Autodesk Fusion 360 part; units mm, degrees
(part 5 of 7)
  spline S1395 degree 3 poles (51.3844, 45.9927) (51.2286, 46.0826) (51.0616, 46.1518) (50.8878, 46.1984) knots 0 0 0 0 1 1 1 1
  line L412 (26.6361, 48.608) -> (26.6361, 48.608)
  spline S1396 degree 3 poles (26.7927, 46.8149) (27.1126, 46.8435) (27.393, 47.0404) (27.5285, 47.3316) knots 0 0 0 0 1 1 1 1
  spline S1397 degree 3 poles (44.8618, 45.1809) (44.5277, 45.1809) (44.2072, 45.0481) (43.9709, 44.8119) knots 0 0 0 0 1 1 1 1
  spline S1398 degree 3 poles (52.4144, 44.2088) (52.4145, 44.3889) (52.3911, 44.5682) (52.3446, 44.7421) knots 0 0 0 0 1 1 1 1
  spline S1399 degree 3 poles (45.7533, 44.8119) (45.9895, 44.5756) (46.1222, 44.2551) (46.1222, 43.921) knots 0 0 0 0 1 1 1 1
  spline S1400 degree 3 poles (25.4878, 46.7012) (25.1676, 46.6732) (24.8568, 46.8182) (24.6724, 47.0815) knots 0 0 0 0 1 1 1 1
  line L413 (30.6519, 45.0444) -> (31.9567, 45.1586)
  spline S1401 degree 3 poles (24.6724, 47.0815) (24.8568, 46.8182) (25.1676, 46.6732) (25.4878, 46.7012) knots 0 0 0 0 1 1 1 1
  spline S1402 degree 3 poles (29.8359, 45.4253) (30.0203, 45.1616) (30.3314, 45.0164) (30.6519, 45.0444) knots 0 0 0 0 1 1 1 1
  spline S1403 degree 3 poles (50.8878, 46.1984) (50.7139, 46.245) (50.5346, 46.2686) (50.3545, 46.2686) knots 0 0 0 0 1 1 1 1
  spline S1404 degree 3 poles (26.6361, 48.608) (26.9561, 48.6355) (27.2664, 48.4904) (27.4505, 48.2272) knots 0 0 0 0 1 1 1 1
  spline S1405 degree 3 poles (52.3446, 44.7421) (52.2979, 44.916) (52.2285, 45.0829) (52.1384, 45.2387) knots 0 0 0 0 1 1 1 1
  spline S1406 degree 3 poles (43.9709, 44.8119) (43.7347, 44.5756) (43.602, 44.2551) (43.602, 43.921) knots 0 0 0 0 1 1 1 1
  spline S1407 degree 3 poles (43.9709, 43.0301) (43.7347, 43.2664) (43.602, 43.5868) (43.602, 43.921) knots 0 0 0 0 1 1 1 1
  spline S1408 degree 3 poles (43.602, 43.921) (43.602, 44.2551) (43.7347, 44.5756) (43.9709, 44.8119) knots 0 0 0 0 1 1 1 1
  spline S1409 degree 3 poles (108.6569, 74.2401) (108.9265, 73.999) (109.0957, 73.6656) (109.1313, 73.3057) knots 0 0 0 0 1 1 1 1
  line L414 (109.1313, 73.3057) -> (109.0982, 72.3565)
  line L415 (109.0982, 72.3565) -> (115.5945, 72.1296)
  line L416 (115.5945, 72.1296) -> (115.6275, 73.0789)
  line L417 (105.1589, 75.596) -> (106.0767, 74.6633)
  spline S1410 degree 3 poles (24.6724, 47.0815) (24.4883, 47.3449) (24.4585, 47.6864) (24.5944, 47.9776) knots 0 0 0 0 1 1 1 1
  line L418 (26.7927, 46.8149) -> (25.4878, 46.7012)
  spline S1411 degree 3 poles (32.6926, 45.6754) (32.8282, 45.9665) (32.7984, 46.3077) (32.6145, 46.571) knots 0 0 0 0 1 1 1 1
  line L419 (106.0767, 74.6633) -> (107.6761, 74.6075)
  line L420 (25.3307, 48.4938) -> (26.6361, 48.608)
  spline S1412 degree 3 poles (44.8618, 42.6611) (44.5277, 42.6611) (44.2072, 42.7938) (43.9709, 43.0301) knots 0 0 0 0 1 1 1 1
  spline S1413 degree 3 poles (27.4505, 48.2272) (27.2664, 48.4904) (26.9561, 48.6355) (26.6361, 48.608) knots 0 0 0 0 1 1 1 1
  spline S1414 degree 3 poles (29.7579, 46.3219) (29.6219, 46.0305) (29.6516, 45.6888) (29.8359, 45.4253) knots 0 0 0 0 1 1 1 1
  spline S1415 degree 3 poles (31.9567, 45.1586) (32.2766, 45.1872) (32.5571, 45.3842) (32.6926, 45.6754) knots 0 0 0 0 1 1 1 1
  spline S1416 degree 3 poles (63.315, 46.2438) (63.315, 46.578) (63.4477, 46.8984) (63.6839, 47.1347) knots 0 0 0 0 1 1 1 1
  spline S1417 degree 3 poles (32.6145, 46.571) (32.4305, 46.8341) (32.1201, 46.9793) (31.8001, 46.9518) knots 0 0 0 0 1 1 1 1
  spline S1418 degree 3 poles (51.8113, 45.6656) (51.6839, 45.7928) (51.5404, 45.9028) (51.3844, 45.9927) knots 0 0 0 0 1 1 1 1
  spline S1419 degree 3 poles (52.1384, 45.2387) (52.0485, 45.3947) (51.9385, 45.5382) (51.8113, 45.6656) knots 0 0 0 0 1 1 1 1
  line L421 (43.4733, 69.0828) -> (43.7141, 64.4892)
  line L422 (101.5374, 58.7118) -> (104.5657, 58.6064)
  line L423 (101.6982, 63.3095) -> (101.5374, 58.7118)
  line L424 (118.201, 72.989) -> (118.3612, 77.5866)
  spline S1420 degree 3 poles (107.0823, 57.6178) (107.4439, 57.6226) (107.7941, 57.4915) (108.0637, 57.2504) knots 0 0 0 0 1 1 1 1
  line L425 (110.2553, 62.51) -> (110.2904, 63.5094)
  line L426 (118.3612, 77.5866) -> (115.7877, 77.676)
  line L427 (110.8485, 79.4997) -> (110.8836, 80.4991)
  line L428 (115.2348, 61.8362) -> (110.7374, 61.9927)
  line L429 (46.0049, 69.6962) -> (46.0297, 69.2166)
  line L430 (115.828, 78.8258) -> (111.3306, 78.9824)
  line L431 (104.2561, 63.2201) -> (101.6982, 63.3095)
  spline S1421 degree 3 poles (107.6761, 74.6075) (108.0375, 74.6121) (108.3875, 74.481) (108.6569, 74.2401) knots 0 0 0 0 1 1 1 1
  line L432 (115.0343, 56.0892) -> (117.6078, 55.9998)
  line L433 (46.0297, 69.2166) -> (43.4733, 69.0828)
  line L434 (43.7141, 64.4892) -> (46.7398, 64.6474)
  line L435 (59.9596, 63.1875) -> (59.7188, 67.781)
  line L436 (46.7398, 64.6474) -> (47.7356, 63.7983)
  line L437 (110.2904, 63.5094) -> (109.8077, 64.0267)
  spline S1422 degree 3 poles (110.7374, 61.9927) (110.6043, 61.9961) (110.4782, 62.0529) (110.3875, 62.1504) knots 0 0 0 0 1 1 1 1
  line L438 (104.8111, 64.2014) -> (104.2732, 63.6996)
  line L439 (51.4899, 70.5044) -> (46.4969, 70.2424)
  line L440 (59.7188, 67.781) -> (57.1474, 67.6461)
  line L441 (50.8971, 62.7126) -> (50.9467, 61.7638)
  line L442 (102.1307, 75.7015) -> (105.1589, 75.596)
  spline S1423 degree 3 poles (49.3334, 63.882) (49.6932, 63.9184) (50.0535, 63.8185) (50.3432, 63.602) knots 0 0 0 0 1 1 1 1
  line L443 (52.0676, 69.0326) -> (52.0154, 70.031)
  line L444 (115.7877, 77.676) -> (115.828, 78.8258)
  spline S1424 degree 3 poles (50.3432, 63.602) (50.6327, 63.3853) (50.8304, 63.068) (50.8971, 62.7126) knots 0 0 0 0 1 1 1 1
  line L445 (105.4834, 57.6736) -> (107.0823, 57.6178)
  line L446 (115.0007, 55.1399) -> (115.0343, 56.0892)
  line L447 (47.7356, 63.7983) -> (49.3334, 63.882)
  line L448 (57.3882, 63.0526) -> (59.9596, 63.1875)
  line L449 (115.6275, 73.0789) -> (118.201, 72.989)
  spline S1425 degree 3 poles (52.5932, 68.5593) (52.4604, 68.5509) (52.3298, 68.5963) (52.2309, 68.6854) knots 0 0 0 0 1 1 1 1
  line L450 (57.1474, 67.6461) -> (57.0869, 68.7949)
  line L451 (52.3797, 53.5276) -> (47.3862, 53.2656)
  line L452 (52.0154, 70.031) -> (51.4899, 70.5044)
  spline S1426 degree 3 poles (52.2309, 68.6854) (52.132, 68.7744) (52.0731, 68.8996) (52.0676, 69.0326) knots 0 0 0 0 1 1 1 1
  line L453 (104.5657, 58.6064) -> (105.4834, 57.6736)
  line L454 (47.3862, 53.2656) -> (46.8943, 52.7194)
  line L455 (57.0869, 68.7949) -> (52.5932, 68.5593)
  line L456 (46.4969, 70.2424) -> (46.0049, 69.6962)
  line L457 (117.768, 60.597) -> (115.1945, 60.6869)
  line L458 (108.538, 56.3161) -> (108.505, 55.3668)
  spline S1427 degree 3 poles (111.3306, 78.9824) (111.1976, 78.9857) (111.0715, 79.0426) (110.9808, 79.14) knots 0 0 0 0 1 1 1 1
  line L459 (110.8836, 80.4991) -> (110.401, 81.0164)
  line L460 (115.1945, 60.6869) -> (115.2348, 61.8362)
  line L461 (108.505, 55.3668) -> (115.0007, 55.1399)
  spline S1428 degree 3 poles (110.3875, 62.1504) (110.2969, 62.2476) (110.2493, 62.3772) (110.2553, 62.51) knots 0 0 0 0 1 1 1 1
  line L462 (110.401, 81.0164) -> (105.4044, 81.1911)
  line L463 (104.2732, 63.6996) -> (104.2561, 63.2201)
  line L464 (109.8077, 64.0267) -> (104.8111, 64.2014)
  line L465 (57.4378, 62.1039) -> (57.3882, 63.0526)
  line L466 (50.9467, 61.7638) -> (57.4378, 62.1039)
  spline S1429 degree 3 poles (110.9808, 79.14) (110.8902, 79.2373) (110.8425, 79.3669) (110.8485, 79.4997) knots 0 0 0 0 1 1 1 1
  line L467 (117.6078, 55.9998) -> (117.768, 60.597)
  spline S1430 degree 3 poles (108.0637, 57.2504) (108.3332, 57.0094) (108.5025, 56.6759) (108.538, 56.3161) knots 0 0 0 0 1 1 1 1
  line L468 (60.849, 46.2108) -> (60.6082, 50.8043)
  line L469 (52.3797, 53.5276) -> (52.9053, 53.0543)
  line L470 (44.604, 47.5125) -> (47.6296, 47.6706)
  spline S1431 degree 3 poles (52.9575, 52.0559) (52.963, 51.9229) (53.0218, 51.7977) (53.1208, 51.7086) knots 0 0 0 0 1 1 1 1
  line L471 (52.9053, 53.0543) -> (52.9575, 52.0559)
  line L472 (50.2233, 46.9053) -> (48.6254, 46.8216)
  spline S1432 degree 3 poles (51.2325, 46.6252) (50.943, 46.8416) (50.5829, 46.9416) (50.2233, 46.9053) knots 0 0 0 0 1 1 1 1
  line L473 (25.9297, 42.6239) -> (26.3307, 38.0412)
  line L474 (30.3738, 37.4919) -> (31.9681, 37.6315)
  line L475 (29.3491, 38.3053) -> (30.3738, 37.4919)
  line L476 (60.6082, 50.8043) -> (60.849, 46.2108)
  line L477 (28.438, 43.3252) -> (28.4799, 42.8472)
  line L478 (33.892, 44.3246) -> (28.9109, 43.8884)
  line L479 (48.6254, 46.8216) -> (47.6296, 47.6706)
  line L480 (28.4799, 42.8472) -> (25.9297, 42.6239)
  line L481 (47.3862, 53.2656) -> (52.3797, 53.5276)
  line L482 (47.6296, 47.6706) -> (44.604, 47.5125)
  line L483 (46.8943, 52.7194) -> (47.3862, 53.2656)
  line L484 (51.8361, 44.7871) -> (51.7865, 45.7359)
  line L485 (40.0461, 37.0832) -> (42.6113, 37.3074)
  line L486 (44.3632, 52.106) -> (46.9196, 52.2399)
  line L487 (42.6113, 37.3074) -> (42.2108, 41.8901)
  line L488 (33.6537, 35.5701) -> (40.1293, 36.137)
  line L489 (26.3307, 38.0412) -> (29.3491, 38.3053)
  line L490 (39.6456, 41.6658) -> (39.5454, 42.8115)
  line L491 (39.5454, 42.8115) -> (35.0624, 42.4193)
  spline S1433 degree 3 poles (35.0624, 42.4193) (34.9301, 42.4062) (34.798, 42.447) (34.6961, 42.5324) knots 0 0 0 0 1 1 1 1
  spline S1434 degree 3 poles (34.6961, 42.5324) (34.5942, 42.618) (34.5311, 42.7409) (34.5209, 42.8735) knots 0 0 0 0 1 1 1 1
  line L492 (34.4335, 43.8698) -> (33.892, 44.3246)
  spline S1435 degree 3 poles (50.2233, 46.9053) (50.5829, 46.9416) (50.943, 46.8416) (51.2325, 46.6252) knots 0 0 0 0 1 1 1 1
  line L493 (58.2776, 46.0759) -> (60.849, 46.2108)
  line L494 (52.9053, 53.0543) -> (52.3797, 53.5276)
  line L495 (58.0367, 50.6694) -> (60.6082, 50.8043)
  line L496 (58.3272, 45.1271) -> (51.8361, 44.7871)
  line L497 (44.604, 47.5125) -> (44.3632, 52.106)
  line L498 (28.9109, 43.8884) -> (28.438, 43.3252)
  line L499 (46.9196, 52.2399) -> (46.8943, 52.7194)
  spline S1436 degree 3 poles (51.7865, 45.7359) (51.7197, 46.0912) (51.522, 46.4086) (51.2325, 46.6252) knots 0 0 0 0 1 1 1 1
  line L500 (57.9768, 51.8182) -> (53.483, 51.5825)
  spline S1437 degree 3 poles (31.9681, 37.6315) (32.3263, 37.6801) (32.6898, 37.5925) (32.9866, 37.386) knots 0 0 0 0 1 1 1 1
  line L501 (40.1293, 36.137) -> (40.0461, 37.0832)
  line L502 (44.3632, 52.106) -> (44.604, 47.5125)
  line L503 (33.5711, 36.5168) -> (33.6537, 35.5701)
  spline S1438 degree 3 poles (32.9866, 37.386) (33.2834, 37.1796) (33.4919, 36.8695) (33.5711, 36.5168) knots 0 0 0 0 1 1 1 1
  line L504 (34.5209, 42.8735) -> (34.4335, 43.8698)
  spline S1439 degree 3 poles (51.2325, 46.6252) (51.522, 46.4086) (51.7197, 46.0912) (51.7865, 45.7359) knots 0 0 0 0 1 1 1 1
  line L505 (58.2776, 46.0759) -> (58.3272, 45.1271)
  line L506 (51.7865, 45.7359) -> (51.8361, 44.7871)
  line L507 (52.9575, 52.0559) -> (52.9053, 53.0543)
  spline S1440 degree 3 poles (53.1208, 51.7086) (53.2197, 51.6196) (53.3502, 51.5742) (53.483, 51.5825) knots 0 0 0 0 1 1 1 1
  spline S1441 degree 3 poles (53.1208, 51.7086) (53.0218, 51.7977) (52.963, 51.9229) (52.9575, 52.0559) knots 0 0 0 0 1 1 1 1
  line L508 (53.483, 51.5825) -> (57.9768, 51.8182)
  line L509 (42.2108, 41.8901) -> (39.6456, 41.6658)
  line L510 (46.9196, 52.2399) -> (44.3632, 52.106)
  line L511 (51.8361, 44.7871) -> (58.3272, 45.1271)
  line L512 (58.0367, 50.6694) -> (57.9768, 51.8182)
  line L513 (60.849, 46.2108) -> (58.2776, 46.0759)
  line L514 (57.9768, 51.8182) -> (58.0367, 50.6694)
  spline S1442 degree 3 poles (53.483, 51.5825) (53.3502, 51.5742) (53.2197, 51.6196) (53.1208, 51.7086) knots 0 0 0 0 1 1 1 1
  line L515 (46.8943, 52.7194) -> (46.9196, 52.2399)
  line L516 (48.6254, 46.8216) -> (50.2233, 46.9053)
  line L517 (47.6296, 47.6706) -> (48.6254, 46.8216)
  line L518 (60.6082, 50.8043) -> (58.0367, 50.6694)
  line L519 (58.3272, 45.1271) -> (58.2776, 46.0759)
  line L520 (82.8492, 51.5396) -> (82.7686, 46.9404)
  spline S1443 degree 3 poles (73.2301, 53.5886) (73.136, 53.6826) (73.0836, 53.8106) (73.0849, 53.9436) knots 0 0 0 0 1 1 1 1
  line L521 (91.4192, 50.8901) -> (91.4363, 51.8895)
  line L522 (85.417, 51.9748) -> (85.4087, 51.4947)
  line L523 (80.6602, 52.2936) -> (78.0851, 52.2936)
  line L524 (101.1044, 46.3198) -> (100.9442, 41.7227)
  line L525 (78.0851, 46.7436) -> (78.0851, 47.6934)
  line L526 (72.5852, 55.4438) -> (67.585, 55.4438)
  line L527 (100.9442, 41.7227) -> (103.9724, 41.6167)
  line L528 (114.4075, 38.1503) -> (114.441, 39.0996)
  line L529 (117.1747, 43.6073) -> (114.6012, 43.6972)
  line L530 (114.6012, 43.6972) -> (114.6415, 44.8465)
  line L531 (85.7984, 46.8872) -> (86.7327, 45.971)
  line L532 (85.9461, 52.4858) -> (85.417, 51.9748)
  line L533 (104.8902, 40.684) -> (106.4891, 40.6282)
  line L534 (103.6799, 46.71) -> (103.6629, 46.2304)
  line L535 (67.0651, 54.4439) -> (64.5051, 54.4439)
  line L536 (73.0849, 54.9436) -> (72.5852, 55.4438)
  line L537 (64.5051, 49.8436) -> (67.5349, 49.8436)
  line L538 (64.5051, 54.4439) -> (64.5051, 49.8436)
  line L539 (71.5853, 46.7436) -> (78.0851, 46.7436)
  line L540 (78.0851, 53.4434) -> (73.5851, 53.4434)
  line L541 (78.0851, 52.2936) -> (78.0851, 53.4434)
  line L542 (86.7327, 45.971) -> (88.332, 45.9431)
  line L543 (89.81, 44.6672) -> (89.7935, 43.7174)
  spline S1444 degree 3 poles (91.5577, 50.5325) (91.4653, 50.6282) (91.4154, 50.7571) (91.4192, 50.8901) knots 0 0 0 0 1 1 1 1
  line L544 (103.6629, 46.2304) -> (101.1044, 46.3198)
  line L545 (104.2179, 47.2117) -> (103.6799, 46.71)
  line L546 (107.9117, 38.3771) -> (114.4075, 38.1503)
  spline S1445 degree 3 poles (106.4891, 40.6282) (106.8507, 40.6329) (107.2009, 40.5018) (107.4704, 40.2607) knots 0 0 0 0 1 1 1 1
  spline S1446 degree 3 poles (107.4704, 40.2607) (107.74, 40.0197) (107.9093, 39.6863) (107.9448, 39.3264) knots 0 0 0 0 1 1 1 1
  line L547 (98.964, 49.1077) -> (96.3894, 49.1527)
  line L548 (114.441, 39.0996) -> (117.014, 39.0102)
  spline S1447 degree 3 poles (110.1441, 45.0036) (110.0112, 45.0068) (109.8851, 45.0634) (109.7943, 45.1607) knots 0 0 0 0 1 1 1 1
  line L549 (85.4087, 51.4947) -> (82.8492, 51.5396)
  line L550 (68.4852, 48.9434) -> (70.0851, 48.9434)
  line L551 (82.7686, 46.9404) -> (85.7984, 46.8872)
  line L552 (71.5853, 47.6934) -> (71.5853, 46.7436)
  spline S1448 degree 3 poles (88.332, 45.9431) (88.6935, 45.9541) (89.0459, 45.8291) (89.3196, 45.5927) knots 0 0 0 0 1 1 1 1
  spline S1449 degree 3 poles (89.3196, 45.5927) (89.5931, 45.3565) (89.7681, 45.0262) (89.81, 44.6672) knots 0 0 0 0 1 1 1 1
  line L553 (103.9724, 41.6167) -> (104.8902, 40.684)
  line L554 (107.9448, 39.3264) -> (107.9117, 38.3771)
  line L555 (117.014, 39.0102) -> (117.1747, 43.6073)
  line L556 (109.6966, 46.5198) -> (109.2145, 47.0371)
  line L557 (67.0651, 54.9234) -> (67.0651, 54.4439)
  line L558 (96.2928, 43.6037) -> (96.3093, 44.5535)
  line L559 (96.4096, 50.3025) -> (91.9101, 50.3811)
  line L560 (90.9453, 52.3985) -> (85.9461, 52.4858)
  spline S1450 degree 3 poles (71.0783, 48.6106) (71.3562, 48.3792) (71.5371, 48.0518) (71.5853, 47.6934) knots 0 0 0 0 1 1 1 1
  spline S1451 degree 3 poles (91.9101, 50.3811) (91.7771, 50.3821) (91.65, 50.4367) (91.5577, 50.5325) knots 0 0 0 0 1 1 1 1
  line L561 (89.7935, 43.7174) -> (96.2928, 43.6037)
  line L562 (96.3093, 44.5535) -> (98.8839, 44.5085)
  spline S1452 degree 3 poles (109.7943, 45.1607) (109.7037, 45.258) (109.656, 45.3876) (109.662, 45.5204) knots 0 0 0 0 1 1 1 1
  line L563 (91.4363, 51.8895) -> (90.9453, 52.3985)
  line L564 (96.3894, 49.1527) -> (96.4096, 50.3025)
  line L565 (73.0849, 53.9436) -> (73.0849, 54.9436)
  line L566 (67.585, 55.4438) -> (67.0651, 54.9234)
  line L567 (98.8839, 44.5085) -> (98.964, 49.1077)
  line L568 (80.6602, 47.6934) -> (80.6602, 52.2936)
  line L569 (109.2145, 47.0371) -> (104.2179, 47.2117)
  spline S1453 degree 3 poles (70.0851, 48.9434) (70.4462, 48.9607) (70.8006, 48.842) (71.0783, 48.6106) knots 0 0 0 0 1 1 1 1
  line L570 (67.5349, 49.8436) -> (68.4852, 48.9434)
  line L571 (78.0851, 47.6934) -> (80.6602, 47.6934)
  spline S1454 degree 3 poles (73.5851, 53.4434) (73.4521, 53.4421) (73.3241, 53.4944) (73.2301, 53.5886) knots 0 0 0 0 1 1 1 1
  line L572 (96.3217, 22.9538) -> (97.0829, 21.8893)
  spline S1455 degree 3 poles (95.2588, 76.2513) (95.495, 76.4876) (95.6277, 76.8081) (95.6277, 77.1422) knots 0 0 0 0 1 1 1 1
  line L573 (95.5197, 77.6223) -> (93.3219, 77.661)
  line L574 (110.7958, 18.1474) -> (111.035, 17.4518)
  line L575 (109.662, 45.5204) -> (109.6966, 46.5198)
  line L576 (118.23, 26.2037) -> (117.1959, 26.7081)
  line L577 (111.035, 17.4518) -> (111.4665, 17.2415)
  line L578 (122.3641, 24.1873) -> (123.4932, 26.5019)
  line L579 (94.2252, 28.0475) -> (93.3478, 23.5321)
  spline S1456 degree 3 poles (100.2342, 85.5541) (99.906, 85.226) (99.7216, 84.781) (99.7215, 84.317) knots 0 0 0 0 1 1 1 1
  spline S1457 degree 3 poles (114.5547, 22.4329) (114.6738, 22.3733) (114.8118, 22.3642) (114.9377, 22.4076) knots 0 0 0 0 1 1 1 1
  line L580 (111.035, 17.4518) -> (110.7958, 18.1474)
  line L581 (120.3688, 17.9288) -> (123.2183, 23.7708)
  line L582 (93.3478, 23.5321) -> (96.3217, 22.9538)
  line L583 (96.7383, 27.5592) -> (94.2252, 28.0475)
  line L584 (114.5547, 22.4329) -> (113.6561, 22.8716)
  line L585 (112.9874, 22.6412) -> (113.6561, 22.8716)
  spline S1458 degree 3 poles (100.2342, 83.0793) (100.5624, 82.751) (101.0076, 82.5666) (101.4718, 82.5667) knots 0 0 0 0 1 1 1 1
  line L586 (110.7958, 18.1474) -> (112.9874, 22.6412)
  spline S1459 degree 3 poles (115.2234, 22.6634) (115.1664, 22.5432) (115.0634, 22.451) (114.9377, 22.4076) knots 0 0 0 0 1 1 1 1
  line L587 (111.4665, 17.2415) -> (110.3441, 14.9409)
  line L588 (117.1959, 26.7081) -> (115.2234, 22.6634)
  line L589 (110.3441, 14.9409) -> (111.4665, 17.2415)
  line L590 (110.3441, 14.9409) -> (114.4788, 12.9239)
  spline S1460 degree 3 poles (114.9377, 22.4076) (114.8118, 22.3642) (114.6738, 22.3733) (114.5547, 22.4329) knots 0 0 0 0 1 1 1 1
  line L591 (114.4788, 12.9239) -> (110.3441, 14.9409)
  line L592 (115.8068, 15.6473) -> (114.4788, 12.9239)
  line L593 (113.6561, 22.8716) -> (114.5547, 22.4329)
  spline S1461 degree 3 poles (101.9245, 86.0073) (101.7768, 86.0468) (101.6247, 86.0668) (101.4718, 86.0667) knots 0 0 0 0 1 1 1 1
  spline S1462 degree 3 poles (102.3467, 85.8321) (102.2142, 85.9087) (102.0723, 85.9676) (101.9245, 86.0073) knots 0 0 0 0 1 1 1 1
  line L594 (111.4665, 17.2415) -> (111.035, 17.4518)
  line L595 (123.2183, 23.7708) -> (122.3641, 24.1873)
  line L596 (97.4395, 28.4413) -> (96.8297, 28.03)
  spline S1463 degree 3 poles (95.6277, 77.1422) (95.6276, 77.2745) (95.6067, 77.406) (95.5657, 77.5318) knots 0 0 0 0 1 1 1 1
  line L597 (113.6561, 22.8716) -> (112.9874, 22.6412)
  line L598 (119.5146, 18.3453) -> (120.3688, 17.9288)
  line L599 (112.9874, 22.6412) -> (110.7958, 18.1474)
  spline S1464 degree 3 poles (118.4687, 18.2916) (118.7983, 18.4398) (119.1716, 18.4589) (119.5146, 18.3453) knots 0 0 0 0 1 1 1 1
  line L600 (97.0829, 21.8893) -> (98.6534, 21.5839)
  spline S1465 degree 3 poles (101.4718, 82.5667) (101.9358, 82.5668) (102.3808, 82.7512) (102.7089, 83.0793) knots 0 0 0 0 1 1 1 1
  spline S1466 degree 3 poles (99.7215, 84.317) (99.7215, 83.8527) (99.9059, 83.4075) (100.2342, 83.0793) knots 0 0 0 0 1 1 1 1
  line L601 (123.4932, 26.5019) -> (119.3586, 28.5183)
  spline S1467 degree 3 poles (102.7089, 83.0793) (103.0372, 83.4075) (103.2216, 83.8527) (103.2216, 84.317) knots 0 0 0 0 1 1 1 1
  spline S1468 degree 3 poles (117.7339, 17.5448) (117.8767, 17.877) (118.1389, 18.1434) (118.4687, 18.2916) knots 0 0 0 0 1 1 1 1
  spline S1469 degree 3 poles (101.4718, 86.0667) (101.0076, 86.0668) (100.5624, 85.8824) (100.2342, 85.5541) knots 0 0 0 0 1 1 1 1
  spline S1470 degree 3 poles (103.2216, 84.317) (103.2216, 84.4698) (103.2016, 84.622) (103.1621, 84.7696) knots 0 0 0 0 1 1 1 1
  spline S1471 degree 3 poles (98.6534, 21.5839) (98.7952, 21.5632) (98.9331, 21.5216) (99.0627, 21.4603) knots 0 0 0 0 1 1 1 1
  spline S1472 degree 3 poles (95.5657, 77.5318) (95.5516, 77.5626) (95.5363, 77.5928) (95.5197, 77.6223) knots 0 0 0 0 1 1 1 1
  spline S1473 degree 3 poles (99.0627, 21.4603) (99.1921, 21.3993) (99.3117, 21.3194) (99.4177, 21.2232) knots 0 0 0 0 1 1 1 1
  spline S1474 degree 3 poles (102.9875, 85.1918) (102.9109, 85.3242) (102.8172, 85.446) (102.7089, 85.5541) knots 0 0 0 0 1 1 1 1
  spline S1475 degree 3 poles (103.1621, 84.7696) (103.1226, 84.9174) (103.0639, 85.0593) (102.9875, 85.1918) knots 0 0 0 0 1 1 1 1
  line L602 (104.8499, 80.2097) -> (102.2914, 80.2991)
  line L603 (114.6415, 44.8465) -> (110.1441, 45.0036)
  spline S1476 degree 3 poles (102.7089, 85.5541) (102.6009, 85.6622) (102.4791, 85.7557) (102.3467, 85.8321) knots 0 0 0 0 1 1 1 1
  line L604 (105.4044, 81.1911) -> (104.8664, 80.6893)
  line L605 (114.4788, 12.9239) -> (115.8068, 15.6473)
  line L606 (115.8068, 15.6473) -> (117.0321, 16.1067)
  line L607 (104.8664, 80.6893) -> (104.8499, 80.2097)
  line L608 (102.2914, 80.2991) -> (102.1307, 75.7015)
  spline S1477 degree 3 poles (94.3679, 75.8823) (94.702, 75.8823) (95.0225, 76.015) (95.2588, 76.2513) knots 0 0 0 0 1 1 1 1
  line L609 (101.4718, 86.0667) -> (101.4718, 86.0667)
  line L610 (119.3586, 28.5183) -> (118.23, 26.2037)
  line L611 (117.0321, 16.1067) -> (117.7339, 17.5448)
  line L612 (96.8297, 28.03) -> (96.7383, 27.5592)
  spline S1478 degree 3 poles (121.6039, 11.6785) (121.2832, 11.6562) (120.9988, 11.4645) (120.8577, 11.1757) knots 0 0 0 0 1 1 1 1
  spline S1479 degree 3 poles (121.6039, 11.6785) (121.63, 11.6804) (121.6563, 11.681) (121.6825, 11.6806) knots 0 0 0 0 1 1 1 1
  line L613 (106.0865, 17.8978) -> (99.706, 19.138)
  line L614 (109.6734, 22.8546) -> (108.7954, 18.3391)
  line L615 (115.2234, 22.6634) -> (117.1959, 26.7081)
  line L616 (99.706, 19.138) -> (99.8874, 20.0708)
  spline S1480 degree 3 poles (132.2467, 31.0722) (132.379, 30.9957) (132.5008, 30.9022) (132.6089, 30.7941) knots 0 0 0 0 1 1 1 1
  line L617 (118.23, 26.2037) -> (119.3586, 28.5183)
  line L618 (108.7954, 18.3391) -> (106.2679, 18.8305)
  spline S1481 degree 3 poles (114.9377, 22.4076) (115.0634, 22.451) (115.1664, 22.5432) (115.2234, 22.6634) knots 0 0 0 0 1 1 1 1
  line L619 (102.9477, 25.3335) -> (107.365, 24.4746)
  line L620 (121.9016, 9.2094) -> (122.4757, 10.3866)
  spline S1482 degree 3 poles (121.1554, 8.7076) (121.4758, 8.7298) (121.7602, 8.921) (121.9016, 9.2094) knots 0 0 0 0 1 1 1 1
  spline S1483 degree 3 poles (131.8245, 31.2473) (131.9723, 31.2077) (132.1142, 31.1488) (132.2467, 31.0722) knots 0 0 0 0 1 1 1 1
  spline S1484 degree 3 poles (99.8487, 20.4961) (99.8148, 20.6353) (99.7605, 20.7687) (99.6874, 20.8919) knots 0 0 0 0 1 1 1 1
  spline S1485 degree 3 poles (99.8874, 20.0708) (99.8956, 20.2137) (99.8826, 20.357) (99.8487, 20.4961) knots 0 0 0 0 1 1 1 1
  line L621 (125.6832, 15.2519) -> (125.6832, 15.2519)
  line L622 (94.2252, 28.0475) -> (96.7383, 27.5592)
  line L623 (117.7339, 17.5448) -> (117.0321, 16.1067)
  line L624 (117.1959, 26.7081) -> (118.23, 26.2037)
  line L625 (121.6039, 11.6785) -> (121.6039, 11.6785)
  spline S1486 degree 3 poles (120.3477, 9.1014) (120.1677, 9.3676) (120.1433, 9.7095) (120.2836, 9.9985) knots 0 0 0 0 1 1 1 1
  spline S1487 degree 3 poles (132.6089, 30.7941) (132.7172, 30.6861) (132.8108, 30.5643) (132.8875, 30.4319) knots 0 0 0 0 1 1 1 1
  line L626 (124.3629, 13.5719) -> (124.937, 14.7491)
  line L627 (102.743, 26.9014) -> (102.5524, 25.9195)
  spline S1488 degree 3 poles (102.5524, 25.9195) (102.5256, 25.7892) (102.5524, 25.6536) (102.6268, 25.5433) knots 0 0 0 0 1 1 1 1
  spline S1489 degree 3 poles (102.6268, 25.5433) (102.7012, 25.4331) (102.8169, 25.3575) (102.9477, 25.3335) knots 0 0 0 0 1 1 1 1
  spline S1490 degree 3 poles (99.4177, 21.2232) (99.3117, 21.3194) (99.1921, 21.3993) (99.0627, 21.4603) knots 0 0 0 0 1 1 1 1
  line L628 (120.8577, 11.1757) -> (120.2836, 9.9985)
  spline S1491 degree 3 poles (120.2836, 9.9985) (120.1433, 9.7095) (120.1677, 9.3676) (120.3477, 9.1014) knots 0 0 0 0 1 1 1 1
  spline S1492 degree 3 poles (133.0621, 30.0097) (133.1016, 29.862) (133.1216, 29.7099) (133.1215, 29.557) knots 0 0 0 0 1 1 1 1
  spline S1493 degree 3 poles (99.6874, 20.8919) (99.6144, 21.0151) (99.5235, 21.1267) (99.4177, 21.2232) knots 0 0 0 0 1 1 1 1
  line L629 (122.4757, 10.3866) -> (121.9016, 9.2094)
  line L630 (97.0829, 21.8893) -> (96.3217, 22.9538)
  line L631 (120.2836, 9.9985) -> (120.8577, 11.1757)
  spline S1494 degree 3 poles (118.4687, 18.2916) (118.1389, 18.1434) (117.8767, 17.877) (117.7339, 17.5448) knots 0 0 0 0 1 1 1 1
  spline S1495 degree 3 poles (132.8875, 30.4319) (132.9639, 30.2994) (133.0226, 30.1575) (133.0621, 30.0097) knots 0 0 0 0 1 1 1 1
  spline S1496 degree 3 poles (120.3477, 9.1014) (120.5274, 8.8355) (120.8352, 8.6855) (121.1554, 8.7076) knots 0 0 0 0 1 1 1 1
  spline S1497 degree 3 poles (121.9016, 9.2094) (121.7602, 8.921) (121.4758, 8.7298) (121.1554, 8.7076) knots 0 0 0 0 1 1 1 1
  line L632 (102.3477, 27.4874) -> (102.743, 26.9014)
  line L633 (93.3478, 23.5321) -> (94.2252, 28.0475)
  line L634 (96.3217, 22.9538) -> (93.3478, 23.5321)
  line L635 (98.6534, 21.5839) -> (97.0829, 21.8893)
  spline S1498 degree 3 poles (99.0627, 21.4603) (98.9331, 21.5216) (98.7952, 21.5632) (98.6534, 21.5839) knots 0 0 0 0 1 1 1 1
  spline S1499 degree 3 poles (124.937, 14.7491) (125.0781, 15.038) (125.3626, 15.2296) (125.6832, 15.2519) knots 0 0 0 0 1 1 1 1
  line L636 (121.6825, 11.6806) -> (121.6825, 11.6806)
  line L637 (107.1454, 23.346) -> (109.6734, 22.8546)
  line L638 (119.3586, 28.5183) -> (123.4932, 26.5019)
  line L639 (96.8297, 28.03) -> (97.4395, 28.4413)
  line L640 (122.3641, 24.1873) -> (123.2183, 23.7708)
  line L641 (96.7383, 27.5592) -> (96.8297, 28.03)
  spline S1500 degree 3 poles (125.2347, 12.2816) (124.9147, 12.2596) (124.6072, 12.4096) (124.4275, 12.6754) knots 0 0 0 0 1 1 1 1
  spline S1501 degree 3 poles (122.4126, 11.2842) (122.5925, 11.0178) (122.6165, 10.6756) (122.4757, 10.3866) knots 0 0 0 0 1 1 1 1
  spline S1502 degree 3 poles (124.4275, 12.6754) (124.2476, 12.9413) (124.223, 13.283) (124.3629, 13.5719) knots 0 0 0 0 1 1 1 1
  line L642 (107.365, 24.4746) -> (107.1454, 23.346)
  spline S1503 degree 3 poles (122.4757, 10.3866) (122.6165, 10.6756) (122.5925, 11.0178) (122.4126, 11.2842) knots 0 0 0 0 1 1 1 1
  line L643 (117.0321, 16.1067) -> (115.8068, 15.6473)
  spline S1504 degree 3 poles (121.6825, 11.6806) (121.9759, 11.6754) (122.2484, 11.5275) (122.4126, 11.2842) knots 0 0 0 0 1 1 1 1
  spline S1505 degree 3 poles (121.1554, 8.7076) (120.8352, 8.6855) (120.5274, 8.8355) (120.3477, 9.1014) knots 0 0 0 0 1 1 1 1
  spline S1506 degree 3 poles (120.8577, 11.1757) (120.9988, 11.4645) (121.2832, 11.6562) (121.6039, 11.6785) knots 0 0 0 0 1 1 1 1
  spline S1507 degree 3 poles (131.3718, 31.3068) (131.5246, 31.3068) (131.6768, 31.2868) (131.8245, 31.2473) knots 0 0 0 0 1 1 1 1
  line L644 (106.2679, 18.8305) -> (106.0865, 17.8978)
  spline S1508 degree 3 poles (122.4126, 11.2842) (122.2328, 11.5506) (121.9246, 11.7009) (121.6039, 11.6785) knots 0 0 0 0 1 1 1 1
  line L645 (97.4395, 28.4413) -> (102.3477, 27.4874)
  line L646 (70.73, 75.2436) -> (69.42, 75.2436)
  line L647 (64.5051, 66.8436) -> (67.5349, 66.8436)
  spline S1509 degree 3 poles (122.9563, 22.4939) (123.0821, 22.4531) (123.2007, 22.3927) (123.3077, 22.3151) knots 0 0 0 0 1 1 1 1
  spline S1510 degree 3 poles (119.5146, 18.3453) (119.1716, 18.4589) (118.7983, 18.4398) (118.4687, 18.2916) knots 0 0 0 0 1 1 1 1
  spline S1511 degree 3 poles (121.9403, 17.382) (122.0303, 17.2262) (122.0994, 17.0592) (122.146, 16.8854) knots 0 0 0 0 1 1 1 1
  line L648 (71.5853, 64.6934) -> (71.5853, 63.7435)
  line L649 (80.6602, 69.2936) -> (78.0851, 69.2936)
  line L650 (78.0851, 70.4434) -> (73.5851, 70.4434)
  line L651 (71.5853, 63.7435) -> (78.0851, 63.7435)
  line L652 (73.0849, 70.9436) -> (73.0849, 71.9436)
  spline S1512 degree 3 poles (118.6997, 14.8959) (118.3134, 15.2821) (118.0963, 15.8059) (118.0961, 16.3521) knots 0 0 0 0 1 1 1 1
  line L653 (78.0851, 63.7435) -> (78.0851, 64.6934)
  line L654 (87.0293, 62.9684) -> (88.6287, 62.9405)
  line L655 (83.0652, 63.9378) -> (86.095, 63.8846)
  spline S1513 degree 3 poles (122.2163, 16.3521) (122.2162, 16.1722) (122.1926, 15.9931) (122.146, 15.8194) knots 0 0 0 0 1 1 1 1
  spline S1514 degree 3 poles (121.6127, 14.8959) (121.4853, 14.7685) (121.3418, 14.6583) (121.1858, 14.5683) knots 0 0 0 0 1 1 1 1
  line L656 (73.0849, 71.9436) -> (72.5852, 72.4438)
  line L657 (119.7348, 18.2378) -> (119.5146, 18.3453)
  spline S1515 degree 3 poles (121.1858, 14.5683) (121.03, 14.4783) (120.863, 14.4092) (120.6892, 14.3626) knots 0 0 0 0 1 1 1 1
  spline S1516 degree 3 poles (118.0961, 16.3521) (118.0961, 16.8986) (118.3133, 17.4226) (118.6997, 17.8089) knots 0 0 0 0 1 1 1 1
  line L658 (67.0651, 71.9234) -> (67.0651, 71.4438)
  spline S1517 degree 3 poles (120.6892, 18.3422) (120.863, 18.2956) (121.03, 18.2265) (121.1858, 18.1365) knots 0 0 0 0 1 1 1 1
  spline S1518 degree 3 poles (73.5851, 70.4434) (73.4521, 70.4421) (73.3241, 70.4944) (73.2301, 70.5886) knots 0 0 0 0 1 1 1 1
  line L659 (85.7053, 68.4921) -> (83.1458, 68.537)
  spline S1519 degree 3 poles (121.1858, 18.1365) (121.3418, 18.0464) (121.4853, 17.9363) (121.6127, 17.8089) knots 0 0 0 0 1 1 1 1
  line L660 (78.0851, 69.2936) -> (78.0851, 70.4434)
  line L661 (86.095, 63.8846) -> (87.0293, 62.9684)
  spline S1520 degree 3 poles (122.146, 16.8854) (122.1926, 16.7115) (122.2163, 16.5322) (122.2163, 16.3521) knots 0 0 0 0 1 1 1 1
  line L662 (85.7136, 68.9722) -> (85.7053, 68.4921)
  line L663 (86.2428, 69.4832) -> (85.7136, 68.9722)
  spline S1521 degree 3 poles (121.9403, 15.3222) (121.8502, 15.1664) (121.7401, 15.0231) (121.6127, 14.8959) knots 0 0 0 0 1 1 1 1
  line L664 (67.0651, 71.4438) -> (64.5051, 71.4438)
  spline S1522 degree 3 poles (88.6287, 62.9405) (88.9901, 62.9515) (89.3425, 62.8265) (89.6162, 62.5901) knots 0 0 0 0 1 1 1 1
  spline S1523 degree 3 poles (123.4581, 20.4046) (123.2218, 20.1683) (122.9013, 20.0356) (122.5672, 20.0356) knots 0 0 0 0 1 1 1 1
  spline S1524 degree 3 poles (121.6127, 17.8089) (121.7401, 17.6815) (121.8502, 17.538) (121.9403, 17.382) knots 0 0 0 0 1 1 1 1
  line L665 (78.0851, 64.6934) -> (80.6602, 64.6934)
  spline S1525 degree 3 poles (70.0851, 65.9434) (70.4462, 65.9607) (70.8006, 65.842) (71.0783, 65.6106) knots 0 0 0 0 1 1 1 1
  spline S1526 degree 3 poles (73.2301, 70.5886) (73.136, 70.6826) (73.0836, 70.8106) (73.0849, 70.9436) knots 0 0 0 0 1 1 1 1
  line L666 (72.5852, 72.4438) -> (67.585, 72.4438)
  line L667 (80.6602, 64.6934) -> (80.6602, 69.2936)
  spline S1527 degree 3 poles (121.6763, 20.4046) (121.6592, 20.4407) (121.6438, 20.4776) (121.6303, 20.5152) knots 0 0 0 0 1 1 1 1
  line L668 (83.1458, 68.537) -> (83.0652, 63.9378)
  spline S1528 degree 3 poles (71.0783, 65.6106) (71.3562, 65.3792) (71.5371, 65.0518) (71.5853, 64.6934) knots 0 0 0 0 1 1 1 1
  line L669 (96.7062, 67.2999) -> (92.2067, 67.3785)
  spline S1529 degree 3 poles (122.146, 15.8194) (122.0995, 15.6454) (122.0303, 15.4782) (121.9403, 15.3222) knots 0 0 0 0 1 1 1 1
  line L670 (64.5051, 71.4438) -> (64.5051, 66.8436)
  spline S1530 degree 3 poles (118.6997, 17.8089) (118.9985, 18.0448) (119.3567, 18.1932) (119.7348, 18.2378) knots 0 0 0 0 1 1 1 1
  line L671 (67.5349, 66.8436) -> (68.4852, 65.9434)
  spline S1531 degree 3 poles (123.3077, 22.3151) (123.4147, 22.2375) (123.5089, 22.1435) (123.5867, 22.0365) knots 0 0 0 0 1 1 1 1
  spline S1532 degree 3 poles (120.1559, 14.2923) (119.6097, 14.2925) (119.0859, 14.5096) (118.6997, 14.8959) knots 0 0 0 0 1 1 1 1
  spline S1533 degree 3 poles (120.6892, 14.3626) (120.5153, 14.316) (120.336, 14.2923) (120.1559, 14.2923) knots 0 0 0 0 1 1 1 1
  spline S1534 degree 3 poles (122.6214, 22.5471) (122.7349, 22.5445) (122.8476, 22.5266) (122.9563, 22.4939) knots 0 0 0 0 1 1 1 1
  spline S1535 degree 3 poles (71.5093, 74.7935) (71.3486, 75.072) (71.0515, 75.2435) (70.73, 75.2436) knots 0 0 0 0 1 1 1 1
  line L672 (67.585, 72.4438) -> (67.0651, 71.9234)
  line L673 (121.6303, 20.5152) -> (120.5776, 18.3567)
  line L674 (123.4932, 26.5019) -> (122.3641, 24.1873)
  spline S1536 degree 3 poles (120.5776, 18.3567) (120.6149, 18.3529) (120.6522, 18.348) (120.6892, 18.3422) knots 0 0 0 0 1 1 1 1
  line L675 (68.4852, 65.9434) -> (70.0851, 65.9434)
  line L676 (123.2183, 23.7708) -> (122.6214, 22.5471)
  spline S1537 degree 3 poles (123.827, 21.2955) (123.827, 20.9614) (123.6943, 20.6409) (123.4581, 20.4046) knots 0 0 0 0 1 1 1 1
  spline S1538 degree 3 poles (122.5672, 20.0356) (122.233, 20.0356) (121.9126, 20.1683) (121.6763, 20.4046) knots 0 0 0 0 1 1 1 1
  spline S1539 degree 3 poles (123.5867, 22.0365) (123.6644, 21.9295) (123.7247, 21.8109) (123.7655, 21.6851) knots 0 0 0 0 1 1 1 1
  spline S1540 degree 3 poles (123.7655, 21.6851) (123.8064, 21.5593) (123.8271, 21.4278) (123.827, 21.2955) knots 0 0 0 0 1 1 1 1
  spline S1541 degree 3 poles (71.5093, 73.8938) (71.67, 74.1722) (71.67, 74.5151) (71.5093, 74.7935) knots 0 0 0 0 1 1 1 1
  line L677 (12.4519, 79.7069) -> (12.4519, 79.7069)
  spline S1542 degree 3 poles (31.9045, 46.9549) (32.1885, 46.9462) (32.4517, 46.8039) (32.6145, 46.571) knots 0 0 0 0 1 1 1 1
  line L678 (30.4948, 46.8376) -> (31.8001, 46.9518)
  spline S1543 degree 3 poles (43.9735, 78.7654) (44.2098, 78.5291) (44.3425, 78.2086) (44.3425, 77.8745) knots 0 0 0 0 1 1 1 1
  spline S1544 degree 3 poles (43.0826, 79.1343) (43.4168, 79.1343) (43.7372, 79.0016) (43.9735, 78.7654) knots 0 0 0 0 1 1 1 1
  spline S1545 degree 3 poles (43.9735, 76.9836) (43.7373, 76.7471) (43.4168, 76.6142) (43.0826, 76.6141) knots 0 0 0 0 1 1 1 1
  spline S1546 degree 3 poles (42.1917, 76.9836) (41.9555, 77.2199) (41.8227, 77.5403) (41.8228, 77.8745) knots 0 0 0 0 1 1 1 1
  line L679 (31.9567, 45.1586) -> (30.6519, 45.0444)
  spline S1547 degree 3 poles (9.5973, 45.7627) (9.4617, 45.4717) (9.1813, 45.275) (8.8615, 45.2465) knots 0 0 0 0 1 1 1 1
  spline S1548 degree 3 poles (89.8984, 75.4545) (89.7425, 75.3645) (89.5756, 75.2954) (89.4017, 75.2488) knots 0 0 0 0 1 1 1 1
  spline S1549 degree 3 poles (86.8086, 77.2383) (86.8085, 77.7847) (87.0254, 78.3087) (87.4117, 78.6951) knots 0 0 0 0 1 1 1 1
  spline S1550 degree 3 poles (88.8684, 75.1785) (88.3221, 75.1784) (87.7981, 75.3953) (87.4117, 75.7816) knots 0 0 0 0 1 1 1 1
  spline S1551 degree 3 poles (87.4117, 75.7816) (87.0254, 76.168) (86.8085, 76.692) (86.8086, 77.2383) knots 0 0 0 0 1 1 1 1
  spline S1552 degree 3 poles (30.6519, 45.0444) (30.3314, 45.0164) (30.0203, 45.1616) (29.8359, 45.4253) knots 0 0 0 0 1 1 1 1
  spline S1553 degree 3 poles (87.4117, 78.6951) (87.798, 79.0815) (88.322, 79.2986) (88.8684, 79.2987) knots 0 0 0 0 1 1 1 1
  spline S1554 degree 3 poles (88.8684, 79.2987) (89.0485, 79.2986) (89.2278, 79.275) (89.4017, 79.2284) knots 0 0 0 0 1 1 1 1
  line L680 (7.3995, 46.9255) -> (8.7044, 47.0397)
  spline S1555 degree 3 poles (89.4017, 79.2284) (89.5756, 79.1816) (89.7425, 79.1123) (89.8984, 79.0222) knots 0 0 0 0 1 1 1 1
  spline S1556 degree 3 poles (90.3252, 78.6951) (90.3521, 78.6623) (90.3779, 78.6287) (90.4027, 78.5943) knots 0 0 0 0 1 1 1 1
  spline S1557 degree 3 poles (89.8984, 79.0222) (90.0543, 78.9323) (90.1978, 78.8223) (90.3252, 78.6951) knots 0 0 0 0 1 1 1 1
  line L681 (90.4027, 78.5943) -> (90.4038, 78.662)
  line L682 (87.3259, 79.9658) -> (86.3916, 80.882)
  line L683 (86.3916, 80.882) -> (83.3623, 80.9353)
  line L684 (86.002, 85.4895) -> (86.0102, 85.9696)
  spline S1558 degree 3 poles (90.4038, 78.662) (90.3618, 79.0211) (90.1866, 79.3514) (89.9128, 79.5875) knots 0 0 0 0 1 1 1 1
  spline S1559 degree 3 poles (11.2143, 79.1943) (11.5425, 79.5225) (11.9877, 79.7069) (12.4519, 79.7069) knots 0 0 0 0 1 1 1 1
  spline S1560 degree 3 poles (11.2143, 76.7195) (10.8862, 77.0476) (10.7018, 77.4926) (10.7017, 77.9566) knots 0 0 0 0 1 1 1 1
  spline S1561 degree 3 poles (90.3252, 75.7816) (90.1978, 75.6543) (90.0543, 75.5444) (89.8984, 75.4545) knots 0 0 0 0 1 1 1 1
  line L685 (88.9258, 79.9379) -> (87.3259, 79.9658)
  line L686 (83.4424, 85.5345) -> (86.002, 85.4895)
  spline S1562 degree 3 poles (14.1423, 78.4098) (14.1818, 78.262) (14.2018, 78.1096) (14.2017, 77.9566) knots 0 0 0 0 1 1 1 1
  spline S1563 degree 3 poles (44.3425, 77.8745) (44.3425, 77.5403) (44.2098, 77.2199) (43.9735, 76.9836) knots 0 0 0 0 1 1 1 1
  spline S1564 degree 3 poles (101.9245, 86.0073) (102.0723, 85.9676) (102.2142, 85.9087) (102.3467, 85.8321) knots 0 0 0 0 1 1 1 1
  spline S1565 degree 3 poles (102.3467, 85.8321) (102.4791, 85.7557) (102.6009, 85.6622) (102.7089, 85.5541) knots 0 0 0 0 1 1 1 1
  line L687 (31.8523, 46.9549) -> (31.8523, 46.9549)
  spline S1566 degree 3 poles (101.4718, 86.0667) (101.6247, 86.0668) (101.7768, 86.0468) (101.9245, 86.0073) knots 0 0 0 0 1 1 1 1
  spline S1567 degree 3 poles (6.6626, 46.4087) (6.7983, 46.7002) (7.0792, 46.8972) (7.3995, 46.9255) knots 0 0 0 0 1 1 1 1
  spline S1568 degree 3 poles (102.9875, 85.1918) (103.0639, 85.0593) (103.1226, 84.9174) (103.1621, 84.7696) knots 0 0 0 0 1 1 1 1
  spline S1569 degree 3 poles (102.7089, 85.5541) (102.8172, 85.446) (102.9109, 85.3242) (102.9875, 85.1918) knots 0 0 0 0 1 1 1 1
  spline S1570 degree 3 poles (12.4519, 76.2069) (11.9877, 76.2068) (11.5425, 76.3912) (11.2143, 76.7195) knots 0 0 0 0 1 1 1 1
  spline S1571 degree 3 poles (41.8228, 77.8745) (41.8227, 78.2086) (41.9555, 78.5291) (42.1917, 78.7654) knots 0 0 0 0 1 1 1 1
  spline S1572 degree 3 poles (6.7412, 45.5126) (6.5569, 45.7759) (6.527, 46.1174) (6.6626, 46.4087) knots 0 0 0 0 1 1 1 1
  spline S1573 degree 3 poles (14.2017, 77.9566) (14.2016, 77.4926) (14.0172, 77.0476) (13.6891, 76.7195) knots 0 0 0 0 1 1 1 1
  spline S1574 degree 3 poles (43.0826, 76.6141) (42.7484, 76.6142) (42.4279, 76.7471) (42.1917, 76.9836) knots 0 0 0 0 1 1 1 1
  line L688 (8.7829, 47.0428) -> (8.7829, 47.0428)
  line L689 (83.3623, 80.9353) -> (83.4424, 85.5345)
  spline S1575 degree 3 poles (89.9128, 79.5875) (89.6393, 79.8238) (89.2871, 79.9488) (88.9258, 79.9379) knots 0 0 0 0 1 1 1 1
  spline S1576 degree 3 poles (103.1621, 84.7696) (103.2016, 84.622) (103.2216, 84.4698) (103.2216, 84.317) knots 0 0 0 0 1 1 1 1
  spline S1577 degree 3 poles (29.8359, 45.4253) (29.6516, 45.6888) (29.6219, 46.0305) (29.7579, 46.3219) knots 0 0 0 0 1 1 1 1
  spline S1578 degree 3 poles (89.4017, 75.2488) (89.2278, 75.2021) (89.0485, 75.1785) (88.8684, 75.1785) knots 0 0 0 0 1 1 1 1
  spline S1579 degree 3 poles (103.2216, 84.317) (103.2216, 83.8527) (103.0372, 83.4075) (102.7089, 83.0793) knots 0 0 0 0 1 1 1 1
  spline S1580 degree 3 poles (90.6523, 76.2084) (90.5624, 76.0524) (90.4524, 75.9089) (90.3252, 75.7816) knots 0 0 0 0 1 1 1 1
  line L690 (86.0102, 85.9696) -> (86.5394, 86.4807)
  spline S1581 degree 3 poles (90.8585, 76.705) (90.8118, 76.5312) (90.7425, 76.3642) (90.6523, 76.2084) knots 0 0 0 0 1 1 1 1
  spline S1582 degree 3 poles (7.5561, 45.1323) (7.2361, 45.1045) (6.9255, 45.2495) (6.7412, 45.5126) knots 0 0 0 0 1 1 1 1
  spline S1583 degree 3 poles (29.7579, 46.3219) (29.8938, 46.613) (30.1747, 46.8096) (30.4948, 46.8376) knots 0 0 0 0 1 1 1 1
  spline S1584 degree 3 poles (32.6145, 46.571) (32.7984, 46.3077) (32.8282, 45.9665) (32.6926, 45.6754) knots 0 0 0 0 1 1 1 1
  spline S1585 degree 3 poles (13.9671, 78.832) (14.0437, 78.6996) (14.1026, 78.5576) (14.1423, 78.4098) knots 0 0 0 0 1 1 1 1
  spline S1586 degree 3 poles (13.6891, 76.7195) (13.361, 76.3914) (12.916, 76.207) (12.4519, 76.2069) knots 0 0 0 0 1 1 1 1
  spline S1587 degree 3 poles (31.8523, 46.9549) (31.8697, 46.9554) (31.8871, 46.9554) (31.9045, 46.9549) knots 0 0 0 0 1 1 1 1
  spline S1588 degree 3 poles (10.7017, 77.9566) (10.7016, 78.4208) (10.886, 78.866) (11.2143, 79.1943) knots 0 0 0 0 1 1 1 1
  spline S1589 degree 3 poles (8.7044, 47.0397) (8.7305, 47.0418) (8.7567, 47.0429) (8.7829, 47.0428) knots 0 0 0 0 1 1 1 1
  spline S1590 degree 3 poles (32.6926, 45.6754) (32.5571, 45.3842) (32.2766, 45.1872) (31.9567, 45.1586) knots 0 0 0 0 1 1 1 1
  spline S1591 degree 3 poles (31.8001, 46.9518) (31.8175, 46.9533) (31.8349, 46.9544) (31.8523, 46.9549) knots 0 0 0 0 1 1 1 1
  line L691 (115.5945, 72.1296) -> (114.2307, 72.1771)
  spline S1592 degree 3 poles (100.2342, 85.5541) (100.5624, 85.8824) (101.0076, 86.0668) (101.4718, 86.0667) knots 0 0 0 0 1 1 1 1
  spline S1593 degree 3 poles (64.9645, 81.4417) (65.0903, 81.4009) (65.2089, 81.3406) (65.3159, 81.2629) knots 0 0 0 0 1 1 1 1
  spline S1594 degree 3 poles (114.3284, 71.7177) (114.3284, 71.3836) (114.1957, 71.0631) (113.9594, 70.8268) knots 0 0 0 0 1 1 1 1
  line L692 (115.7877, 77.676) -> (118.3612, 77.5866)
  spline S1595 degree 3 poles (114.2664, 72.1069) (114.3073, 71.9812) (114.3283, 71.8499) (114.3284, 71.7177) knots 0 0 0 0 1 1 1 1
  spline S1596 degree 3 poles (65.5944, 80.9843) (65.6721, 80.8773) (65.7324, 80.7587) (65.7732, 80.6329) knots 0 0 0 0 1 1 1 1
  spline S1597 degree 3 poles (109.6315, 71.9095) (109.6315, 71.7294) (109.6079, 71.5501) (109.5612, 71.3761) knots 0 0 0 0 1 1 1 1
  spline S1598 degree 3 poles (109.0285, 70.4527) (108.9011, 70.3255) (108.7576, 70.2155) (108.6016, 70.1256) knots 0 0 0 0 1 1 1 1
  spline S1599 degree 3 poles (107.5717, 69.8496) (107.0253, 69.8495) (106.5013, 70.0664) (106.1149, 70.4527) knots 0 0 0 0 1 1 1 1
  line L693 (109.1287, 73.2355) -> (109.1313, 73.3057)
  line L694 (112.0303, 72.2541) -> (109.5747, 72.3399)
  spline S1600 degree 3 poles (99.7215, 84.317) (99.7216, 84.781) (99.906, 85.226) (100.2342, 85.5541) knots 0 0 0 0 1 1 1 1
  spline S1601 degree 3 poles (101.4718, 82.5667) (101.0076, 82.5666) (100.5624, 82.751) (100.2342, 83.0793) knots 0 0 0 0 1 1 1 1
  spline S1602 degree 3 poles (65.8352, 80.2438) (65.8354, 79.9095) (65.7026, 79.5888) (65.4663, 79.3524) knots 0 0 0 0 1 1 1 1
  line L695 (110.401, 81.0164) -> (110.8836, 80.4991)
  line L696 (111.3306, 78.9824) -> (115.828, 78.8258)
  spline S1603 degree 3 poles (112.1771, 70.8268) (111.9408, 71.0631) (111.8081, 71.3836) (111.8081, 71.7177) knots 0 0 0 0 1 1 1 1
  spline S1604 degree 3 poles (109.5612, 71.3761) (109.5147, 71.2023) (109.4455, 71.0354) (109.3556, 70.8795) knots 0 0 0 0 1 1 1 1
  spline S1605 degree 3 poles (109.3556, 70.8795) (109.2656, 70.7236) (109.1557, 70.5801) (109.0285, 70.4527) knots 0 0 0 0 1 1 1 1
  spline S1606 degree 3 poles (108.105, 69.9199) (107.9311, 69.8733) (107.7518, 69.8496) (107.5717, 69.8496) knots 0 0 0 0 1 1 1 1
  spline S1607 degree 3 poles (106.1149, 70.4527) (105.7287, 70.8391) (105.5118, 71.3631) (105.5119, 71.9095) knots 0 0 0 0 1 1 1 1
  spline S1608 degree 3 poles (64.5748, 78.9834) (64.2407, 78.9834) (63.9202, 79.1162) (63.6839, 79.3524) knots 0 0 0 0 1 1 1 1
  spline S1609 degree 3 poles (65.4663, 79.3524) (65.2298, 79.116) (64.9092, 78.9833) (64.5748, 78.9834) knots 0 0 0 0 1 1 1 1
  line L697 (107.6761, 74.6075) -> (106.0767, 74.6633)
  line L698 (102.1307, 75.7015) -> (102.2914, 80.2991)
  spline S1610 degree 3 poles (113.9594, 70.8268) (113.7232, 70.5904) (113.4027, 70.4575) (113.0685, 70.4573) knots 0 0 0 0 1 1 1 1
  spline S1611 degree 3 poles (108.6569, 74.2401) (108.3875, 74.481) (108.0375, 74.6121) (107.6761, 74.6075) knots 0 0 0 0 1 1 1 1
  spline S1612 degree 3 poles (108.6016, 73.6933) (108.7576, 73.6034) (108.9011, 73.4934) (109.0285, 73.3662) knots 0 0 0 0 1 1 1 1
  spline S1613 degree 3 poles (110.8485, 79.4997) (110.8425, 79.3669) (110.8902, 79.2373) (110.9808, 79.14) knots 0 0 0 0 1 1 1 1
  line L699 (105.1589, 75.596) -> (102.1307, 75.7015)
  spline S1614 degree 3 poles (108.6016, 70.1256) (108.4458, 70.0356) (108.2788, 69.9665) (108.105, 69.9199) knots 0 0 0 0 1 1 1 1
  line L700 (115.6275, 73.0789) -> (115.5945, 72.1296)
  spline S1615 degree 3 poles (105.5119, 71.9095) (105.5118, 72.4558) (105.7287, 72.9798) (106.1149, 73.3662) knots 0 0 0 0 1 1 1 1
  line L701 (101.4718, 86.0667) -> (101.4718, 86.0667)
  spline S1616 degree 3 poles (108.105, 73.8995) (108.2788, 73.8528) (108.4458, 73.7835) (108.6016, 73.6933) knots 0 0 0 0 1 1 1 1
  spline S1617 degree 3 poles (110.9808, 79.14) (111.0715, 79.0426) (111.1976, 78.9857) (111.3306, 78.9824) knots 0 0 0 0 1 1 1 1
  line L702 (118.201, 72.989) -> (115.6275, 73.0789)
  spline S1618 degree 3 poles (111.8081, 71.7177) (111.8394, 71.9114) (111.9155, 72.0951) (112.0303, 72.2541) knots 0 0 0 0 1 1 1 1
  spline S1619 degree 3 poles (107.5717, 73.9693) (107.7517, 73.9694) (107.931, 73.946) (108.105, 73.8995) knots 0 0 0 0 1 1 1 1
  spline S1620 degree 3 poles (106.1149, 73.3662) (106.5013, 73.7525) (107.0253, 73.9694) (107.5717, 73.9693) knots 0 0 0 0 1 1 1 1
  spline S1621 degree 3 poles (63.315, 80.2438) (63.315, 80.578) (63.4477, 80.8984) (63.6839, 81.1347) knots 0 0 0 0 1 1 1 1
  spline S1622 degree 3 poles (63.6839, 81.1347) (63.9202, 81.371) (64.2407, 81.5037) (64.5748, 81.5037) knots 0 0 0 0 1 1 1 1
  line L703 (104.8499, 80.2097) -> (104.8664, 80.6893)
  spline S1623 degree 3 poles (102.7089, 83.0793) (102.3808, 82.7512) (101.9358, 82.5668) (101.4718, 82.5667) knots 0 0 0 0 1 1 1 1
  spline S1624 degree 3 poles (109.0285, 73.3662) (109.0636, 73.324) (109.097, 73.2804) (109.1287, 73.2355) knots 0 0 0 0 1 1 1 1
  line L704 (106.0767, 74.6633) -> (105.1589, 75.596)
  line L705 (102.2914, 80.2991) -> (104.8499, 80.2097)
  spline S1625 degree 3 poles (100.2342, 83.0793) (99.9059, 83.4075) (99.7215, 83.8527) (99.7215, 84.317) knots 0 0 0 0 1 1 1 1
  line L706 (104.8664, 80.6893) -> (105.4044, 81.1911)
  spline S1626 degree 3 poles (12.9046, 79.647) (13.0524, 79.6074) (13.1943, 79.5487) (13.3268, 79.4723) knots 0 0 0 0 1 1 1 1
  line L707 (105.4044, 81.1911) -> (110.401, 81.0164)
  line L708 (110.8836, 80.4991) -> (110.8485, 79.4997)
  spline S1627 degree 3 poles (109.1313, 73.3057) (109.0957, 73.6656) (108.9265, 73.999) (108.6569, 74.2401) knots 0 0 0 0 1 1 1 1
  line L709 (118.3612, 77.5866) -> (118.201, 72.989)
  line L710 (115.828, 78.8258) -> (115.7877, 77.676)
  spline S1628 degree 3 poles (113.0685, 70.4573) (112.7341, 70.4573) (112.4134, 70.5903) (112.1771, 70.8268) knots 0 0 0 0 1 1 1 1
  spline S1629 degree 3 poles (114.2307, 72.1771) (114.2433, 72.1541) (114.2552, 72.1306) (114.2664, 72.1069) knots 0 0 0 0 1 1 1 1
  line L711 (64.5748, 81.5037) -> (64.5748, 81.5037)
  spline S1630 degree 3 poles (63.6839, 79.3524) (63.4476, 79.5888) (63.3148, 79.9095) (63.315, 80.2438) knots 0 0 0 0 1 1 1 1
  spline S1631 degree 3 poles (109.5747, 72.3399) (109.6087, 72.1988) (109.6278, 72.0545) (109.6315, 71.9095) knots 0 0 0 0 1 1 1 1
  spline S1632 degree 3 poles (65.3159, 81.2629) (65.4228, 81.1852) (65.5168, 81.0912) (65.5944, 80.9843) knots 0 0 0 0 1 1 1 1
  spline S1633 degree 3 poles (64.5748, 81.5037) (64.7072, 81.5036) (64.8387, 81.4827) (64.9645, 81.4417) knots 0 0 0 0 1 1 1 1
  spline S1634 degree 3 poles (65.7732, 80.6329) (65.8142, 80.5073) (65.8351, 80.376) (65.8352, 80.2438) knots 0 0 0 0 1 1 1 1
  spline S1635 degree 3 poles (102.7033, 34.706) (102.5527, 34.9897) (102.2625, 35.1717) (101.9416, 35.1835) knots 0 0 0 0 1 1 1 1
  spline S1636 degree 3 poles (105.3548, 49.5232) (105.1845, 49.2506) (105.1724, 48.9079) (105.3233, 48.6241) knots 0 0 0 0 1 1 1 1
  spline S1637 degree 3 poles (89.3051, 45.0274) (89.1491, 45.1176) (88.982, 45.1869) (88.808, 45.2336) knots 0 0 0 0 1 1 1 1
  spline S1638 degree 3 poles (101.8785, 33.3847) (102.1995, 33.3741) (102.5018, 33.5354) (102.6717, 33.8079) knots 0 0 0 0 1 1 1 1
  spline S1639 degree 3 poles (100.8884, 36.862) (101.2226, 36.8621) (101.5431, 36.995) (101.7793, 37.2315) knots 0 0 0 0 1 1 1 1
  line L712 (100.5695, 33.4307) -> (101.8785, 33.3847)
  spline S1640 degree 3 poles (105.3233, 48.6241) (105.4742, 48.3401) (105.7652, 48.1583) (106.0865, 48.1471) knots 0 0 0 0 1 1 1 1
  spline S1641 degree 3 poles (102.0868, 38.5115) (102.046, 38.6373) (101.9856, 38.7559) (101.908, 38.8629) knots 0 0 0 0 1 1 1 1
  spline S1642 degree 3 poles (89.732, 44.7003) (89.6046, 44.8275) (89.4611, 44.9375) (89.3051, 45.0274) knots 0 0 0 0 1 1 1 1
  spline S1643 degree 3 poles (99.9975, 37.2315) (100.2337, 36.995) (100.5542, 36.8621) (100.8884, 36.862) knots 0 0 0 0 1 1 1 1
  spline S1644 degree 3 poles (103.2665, 50.7971) (103.4368, 51.0696) (103.4489, 51.4124) (103.2981, 51.6962) knots 0 0 0 0 1 1 1 1
  spline S1645 degree 3 poles (106.149, 49.9459) (105.8278, 49.957) (105.525, 49.7959) (105.3548, 49.5232) knots 0 0 0 0 1 1 1 1
  spline S1646 degree 3 poles (102.2222, 56.1311) (102.1153, 56.2089) (101.9969, 56.2694) (101.8713, 56.3104) knots 0 0 0 0 1 1 1 1
  spline S1647 degree 3 poles (100.8884, 39.3822) (100.5542, 39.3823) (100.2338, 39.2495) (99.9975, 39.0133) knots 0 0 0 0 1 1 1 1
  spline S1648 degree 3 poles (12.4519, 79.7069) (12.6048, 79.7068) (12.757, 79.6866) (12.9046, 79.647) knots 0 0 0 0 1 1 1 1
  spline S1649 degree 3 poles (102.1483, 38.1224) (102.1483, 38.2545) (102.1275, 38.3858) (102.0868, 38.5115) knots 0 0 0 0 1 1 1 1
  spline S1650 degree 3 poles (86.8184, 44.7003) (86.432, 44.314) (86.2149, 43.7899) (86.2149, 43.2435) knots 0 0 0 0 1 1 1 1
  spline S1651 degree 3 poles (99.8078, 33.9076) (99.9585, 33.6242) (100.2487, 33.4424) (100.5695, 33.4307) knots 0 0 0 0 1 1 1 1
  spline S1652 degree 3 poles (101.4816, 53.8516) (101.8158, 53.8518) (102.1363, 53.9847) (102.3725, 54.2211) knots 0 0 0 0 1 1 1 1
  spline S1653 degree 3 poles (86.2149, 43.2435) (86.2149, 42.6971) (86.432, 42.1731) (86.8184, 41.7868) knots 0 0 0 0 1 1 1 1
  spline S1654 degree 3 poles (101.908, 38.8629) (101.8301, 38.9698) (101.736, 39.0638) (101.6289, 39.1414) knots 0 0 0 0 1 1 1 1
  spline S1655 degree 3 poles (101.278, 39.3208) (101.1522, 39.3616) (101.0207, 39.3823) (100.8884, 39.3822) knots 0 0 0 0 1 1 1 1
  spline S1656 degree 3 poles (89.809, 44.6) (89.7843, 44.6342) (89.7586, 44.6676) (89.732, 44.7003) knots 0 0 0 0 1 1 1 1